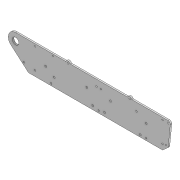
# Autodesk Inventor part: plyta_boczna
Saved by Autodesk Inventor 2020.3 (Build 243373000, 373)
## iProperties
Created: 2021-11-07
Part Number: plyta_boczna
Material: Ogólny
Document SubType Name: Modeling
Designer: patry
Density: 1 g/cm^3
Appearance: Domyślna
Author: patry
Autodesk Inventor part; units mm, degrees
ref_plane "YZ Plane" through (0, 0, 0) normal (1, 0, 0) x (0, 1, 0)
ref_plane "XZ Plane" through (0, 0, 0) normal (0, 1, 0) x (-1, 0, 0)
ref_plane "XY Plane" through (0, 0, 0) normal (0, 0, 1) x (1, 0, 0)
sketch "Szkic1" plane through (0, 0, 0) normal (0, 0, 1) x (1, 0, 0)
  line L0 (-215, -55) -> (215, -55) construction
  line L1 (215, -55) -> (215, 55) construction
  line L2 (215, 55) -> (-215, 55) construction
  line L3 (-215, 55) -> (-215, -55) construction
  line L4 (-215, -55) -> (215, 55) construction
  line L5 (215, -55) -> (-215, 55) construction
  circle A0 centre (-280, 8) radius 41.25 construction
  circle A1 centre (-280, 8) radius 11
  arc A2 (-280, 33) -> (-296.3719, -10.8934) centre (-280, 8) ccw
  line L6 (-280, 33) -> (-111.2284, 33)
  line L7 (-236.8172, -62.5) -> (215, -62.5)
  line L8 (-296.3719, -10.8934) -> (-236.8172, -62.5)
  arc A3 (-296.3719, -10.8934) -> (-280, 33) centre (-280, 8) ccw construction
  circle A4 centre (-200, -120) radius 25 construction
  circle A5 centre (-120, -120) radius 25 construction
  circle A6 centre (-40, -120) radius 25 construction
  circle A7 centre (40, -120) radius 25 construction
  circle A8 centre (120, -120) radius 25 construction
  circle A9 centre (200, -120) radius 25 construction
  line L9 (-120, -120) -> (-40, -120) construction
  line L10 (40, -120) -> (120, -120) construction
  arc A10 (-111.2284, 33) -> (-96.7716, 33) centre (-104, 31) ccw construction
  arc A11 (96.7716, 33) -> (111.2284, 33) centre (104, 31) ccw construction
  line L11 (-96.7716, 33) -> (96.7716, 33)
  line L12 (-111.2284, 33) -> (-96.7716, 33) construction
  arc A12 (-96.7716, 33) -> (-111.2284, 33) centre (-104, 31) ccw
  arc A13 (111.2284, 33) -> (96.7716, 33) centre (104, 31) ccw
  line L13 (111.2284, 33) -> (233.5, 33)
  line L14 (96.7716, 33) -> (111.2284, 33) construction
  arc A14 (240.9621, 24.7471) -> (233.5, 33) centre (233.5, 25.5) ccw
  arc A15 (231.7135, -47.4781) -> (234.1621, -42.6529) centre (226.7, -41.9) ccw
  line L15 (240.9621, 24.7471) -> (234.1621, -42.6529)
  arc A16 (233.5, 33) -> (240.9621, 24.7471) centre (233.5, 25.5) ccw construction
  line L16 (215, -62.5) -> (231.7135, -47.4781)
  arc A17 (234.1621, -42.6529) -> (231.7135, -47.4781) centre (226.7, -41.9) ccw construction
  point P0 (0, 0)
  point P1 (-215, 25.5)
  point P2 (-215, -44.5)
  point P3 (215, 25.5)
  point P4 (215, -44.5)
  point P5 (-252.055, -39.3717)
  point P6 (-80, -120)
  point P7 (80, -120)
  point P8 (-150, -32.735)
  point P9 (-20, -50)
  point P10 (20, -50)
  point P11 (140, -55)
  point P12 (-178.648, -14.42)
  point P13 (160.115, -11.966)
  point P14 (-40.115, -6.966)
  point P15 (40.115, -6.966)
  point P16 (0, -55)
  point P17 (-160, -55)
  point P18 (160, -55)
  point P19 (-154.542, 27.216)
  point P20 (-7.339, 11.921)
  point P21 (7.339, 11.921)
  point P22 (127.339, 6.921)
  dimension "d0" = 430
  dimension "d1" = 110
  dimension "d2" = 63
  dimension "d3" = 65
  dimension "d4" = 82.5
  dimension "d7" = 22
  dimension "d8" = 50
  dimension "d9" = 17.5
  dimension "d10" = 70
  dimension "d11" = 7.5
  dimension "d12" = 7.5
  dimension "d13" = 7.5
  dimension "d15" = 55
  dimension "d16" = 15
  dimension "d17" = 50
  dimension "d18" = 65
  dimension "d21" = 80
  dimension "d26" = 23
  dimension "d27" = 208
  dimension "d28" = 104
  dimension "d29" = 15
  dimension "d30" = 15
  dimension "d31" = 18.5
  dimension "d32" = 67.4
  dimension "d33" = 6.8
  dimension "d34" = 15
  dimension "d35" = 15
  dimension "d38" = 70
  dimension "d39" = 60
  dimension "d40" = 60
  dimension "d41" = 60
  dimension "d43" = 18.315
  dimension "d44" = 39.885
  dimension "d45" = 43.034
  dimension "d46" = 39.885
  dimension "d47" = 39.885
  dimension "d48" = 40
  dimension "d49" = 40
  dimension "d50" = 59.951
  dimension "d52" = 61.921
  dimension "d53" = 12.661
  dimension "d54" = 12.661
  dimension "d55" = 12.661
  dimension "d56" = 61.921
  dimension "d73" = 130
  dimension "d74" = 40.735
  dimension "d75" = 28.648
  dimension "d76" = 4.542
  dimension "d77" = 43.034
  constraints: 34 end point, 20 point on circle, 18 centre point, 13 coincident, 10 horizontal, 8 point on line, 7 horizontal alignment, 5 midpoint, 4 tangent, 2 parallel, 1 perpendicular, 15 other
  measures "d0" distance of L2.end L1.end
  measures "d1" distance of L1.end L0.end
  measures "d2" distance from line of L0 point (-280, 8)
  measures "d3" distance from line of L3 point (-280, 8)
  measures "d4" diameter of A0
  measures "d7" diameter of A1
  measures "d8" diameter of A2
  measures "d9" vertical distance of point (-280, 8) point (-215, 25.5)
  measures "d10" distance of point (-215, -44.5) point (-215, 25.5)
  measures "d11" distance from line of point (215, 25.5) L6
  measures "d12" distance between parallel lines of L7 L0
  measures "d13" distance from line of L8 point (-252.055, -39.372)
  measures "d15" distance of point (-280, 8) point (-252.055, -39.372)
  measures "d16" distance from line of point (-200, -120) L3
  measures "d17" diameter of A4
  measures "d18" distance from line of point (-200, -120) L0
  measures "d21" distance of A4.centre A5.centre
  measures "d26" vertical distance of point (-280, 8) point (-104, 31)
  measures "d27" distance of point (104, 31) point (-104, 31)
  measures "d28" horizontal distance of point (0, 0) point (-104, 31)
  measures "d29" diameter of A10
  measures "d30" diameter of A11
  measures "d31" distance of point (215, 25.5) point (233.5, 25.5)
  measures "d32" vertical distance of point (226.7, -41.9) point (233.5, 25.5)
  measures "d33" horizontal distance of point (233.5, 25.5) point (226.7, -41.9)
  measures "d34" diameter of A14
  measures "d35" diameter of A15
  measures "d38" vertical distance of point (-80, -120) point (-20, -50)
  measures "d39" horizontal distance of point (-20, -50) point (-80, -120)
  measures "d40" horizontal distance of point (80, -120) point (20, -50)
  measures "d41" horizontal distance of point (200, -120) point (140, -55)
  measures "d43" vertical distance of point (-150, -32.735) point (-178.648, -14.42)
  measures "d44" horizontal distance of point (200, -120) point (160.115, -11.966)
  measures "d45" vertical distance of point (-20, -50) point (-40.115, -6.966)
  measures "d46" horizontal distance of point (-40.115, -6.966) point (-80, -120)
  measures "d47" horizontal distance of point (80, -120) point (40.115, -6.966)
  measures "d48" horizontal distance of point (200, -120) point (160, -55)
  measures "d49" horizontal distance of point (-200, -120) point (-160, -55)
  measures "d50" vertical distance of point (-150, -32.735) point (-154.542, 27.216)
  measures "d52" vertical distance of point (-20, -50) point (-7.339, 11.921)
  measures "d53" horizontal distance of point (-7.339, 11.921) point (-20, -50)
  measures "d54" horizontal distance of point (20, -50) point (7.339, 11.921)
  measures "d55" horizontal distance of point (140, -55) point (127.339, 6.921)
  measures "d56" vertical distance of point (140, -55) point (127.339, 6.921)
  measures "d73" horizontal distance of A0.centre point (-150, -32.735)
  measures "d74" vertical distance of A0.centre point (-150, -32.735)
  measures "d75" horizontal distance of point (-150, -32.735) point (-178.648, -14.42)
  measures "d76" horizontal distance of point (-150, -32.735) point (-154.542, 27.216)
  measures "d77" vertical distance of point (160, -55) point (160.115, -11.966)
extrude "Wyciągnięcie proste1" add sketch "Szkic1" along normal blind 5
hole "Otwór1" at (-280, 8, 0) at (-215, 25.5, 0) at (-215, -44.5, 0) at (215, 25.5, 0) at (215, -44.5, 0) at (-252.055, -39.3717, 0) at (-200, -120, 0) at (-120, -120, 0) at (-40, -120, 0) at (40, -120, 0) at (120, -120, 0) at (200, -120, 0) at (-80, -120, 0) at (80, -120, 0) at (-104, 31, 0) at (104, 31, 0) at (226.7, -41.9, 0) at (0, -55, 0) at (-160, -55, 0) at (160, -55, 0) at (-154.542, 27.216, 0) at (-7.339, 11.921, 0) at (7.339, 11.921, 0) at (127.339, 6.921, 0) direction (0, 0, 1) diameter 5 end through all
hole "Otwór2" at (233.5, 25.5, 0) at (-150, -32.735, 0) at (-20, -50, 0) at (20, -50, 0) at (140, -55, 0) at (-178.648, -14.42, 0) at (160.115, -11.966, 0) at (-40.115, -6.966, 0) at (40.115, -6.966, 0) direction (0, 0, 1) diameter 6 end through all
equation "\"d12\" = d11"
equation "\"d13\" = d11"
equation "\"d28\" = 0.5 * d27"
equation "\"d29\" = 2 * d11"
equation "\"d30\" = d29"
equation "\"d34\" = d30"
equation "\"d35\" = d34"
equation "\"d39\" = d37"
equation "\"d40\" = d39"
equation "\"d41\" = d37"
equation "\"d44\" = d47"
equation "\"d47\" = d46"
equation "\"d49\" = d48"
equation "\"d54\" = d53"
equation "\"d55\" = d54"
equation "\"d56\" = d52"
equation "\"d77\" = d45"
equation "\"d37\" = 60"
